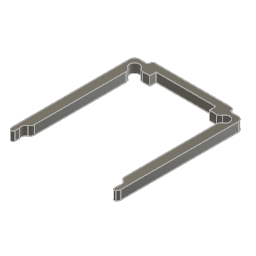
Screen Spacer v4 (Autodesk Fusion 360 design; units mm, degrees)
Autodesk Fusion 360 part; units mm, degrees
sketch "Sketch1" plane through (0, 0, 0) normal (0, 1, 0) x (1, 0, 0)
  line L0 (0, 0) -> (20, 0) construction
  line L1 (20, 0) -> (20, 24) construction
  line L2 (20, 24) -> (0, 24) construction
  line L3 (0, 24) -> (0, 0) construction
  circle A0 centre (0, 24) radius 1.1
  circle A1 centre (20, 24) radius 1.1
  circle A2 centre (20, 0) radius 1.1
  circle A3 centre (0, 0) radius 1.1
  line L4 (-2, 26) -> (22, 26)
  line L5 (22, 26) -> (22, -2)
  line L6 (22, -2) -> (-2, -2)
  line L7 (-2, -2) -> (-2, 26)
  line L8 (0, 24) -> (20, 24)
  line L9 (20, 24) -> (20, 0)
  line L10 (20, 0) -> (0, 0)
  line L11 (0, 0) -> (0, 24)
  dimension "d1" = 24
  dimension "d2" = 20
  dimension "d3" = 2.2
  dimension "d4" = 2
  dimension "d5" = 2
  dimension "d6" = 2
  dimension "d7" = 2
  constraint horizontal L0
  constraint vertical L1
  constraint horizontal L2
  constraint vertical L3
  constraint coincident L0.start L3.end
  constraint coincident L2.end L3.start
  constraint coincident L1.end L2.start
  constraint coincident L0.end L1.start
  constraint equal A0 A3
  constraint equal A0 A1
  constraint equal A1 A2
  constraint horizontal L4
  constraint vertical L5
  constraint horizontal L6
  constraint vertical L7
  constraint horizontal L8
  constraint vertical L9
  constraint horizontal L10
  constraint vertical L11
  measures "d1" distance of L0.start L2.end
  measures "d2" distance of L1.end L2.end
  measures "d3" diameter of A0
  measures "d4" distance of L2 L4
  measures "d5" distance of L1 L5
  measures "d6" distance of L0 L6
  measures "d7" distance of L3 L7
extrude "Extrude1" add sketch "Sketch1" along normal blind 2
fillet "Fillet1" radius 1 8 edges at (1.1, 1, -24) (0, 1, -22.9) (0, 1, -1.1) (18.9, 1, -24) (1.1, 1, 0) (20, 1, -22.9) (20, 1, -1.1) (18.9, 1, 0)
fillet "Fillet2" radius 1 4 edges at (-2, 1, -26) (-2, 1, 2) (22, 1, 2) (22, 1, -26)
extrude "Extrude2" cut 1 faces at (13.6667, 0.6667, 2) along direction (0, 0, -1) up to surface (2 mm away)
fillet "Fillet3" radius 0.4 2 edges at (-1, 1, 2) (21, 1, 2)
sketch "Sketch2" plane through (0, 2, 0) normal (0, 1, 0) x (-1, 0, 0)
  arc A0 (-21, 1.4472) -> (-21.6667, 1.7454) centre (-21.4, 1.4472) ccw
  arc A1 (-21.6667, 1.7454) -> (-22, 1) centre (-21, 1) ccw
  line L0 (-22, 1) -> (-22, -25)
  arc A2 (-22, -25) -> (-21, -26) centre (-21, -25) ccw
  line L1 (-21, -26) -> (1, -26)
  arc A3 (1, -26) -> (2, -25) centre (1, -25) ccw
  line L2 (2, -25) -> (2, 1)
  arc A4 (2, 1) -> (1.6667, 1.7454) centre (1, 1) ccw
  arc A5 (1.6667, 1.7454) -> (1, 1.4472) centre (1.4, 1.4472) ccw
  line L3 (1, 1.4472) -> (1, 0.4583)
  arc A6 (0.5238, -0.9673) -> (1, 0.4583) centre (0, 0) ccw
  arc A7 (0.5238, -0.9673) -> (0, -1.8466) centre (1, -1.8466) ccw
  line L4 (0, -1.8466) -> (0, -22.1534)
  arc A8 (0, -22.1534) -> (0.5238, -23.0327) centre (1, -22.1534) ccw
  arc A9 (-0.9673, -24.5238) -> (0.5238, -23.0327) centre (0, -24) ccw
  arc A10 (-0.9673, -24.5238) -> (-1.8466, -24) centre (-1.8466, -25) ccw
  line L5 (-1.8466, -24) -> (-18.1534, -24)
  arc A11 (-18.1534, -24) -> (-19.0327, -24.5238) centre (-18.1534, -25) ccw
  arc A12 (-20.5238, -23.0327) -> (-19.0327, -24.5238) centre (-20, -24) ccw
  arc A13 (-20.5238, -23.0327) -> (-20, -22.1534) centre (-21, -22.1534) ccw
  line L6 (-20, -22.1534) -> (-20, -1.8466)
  arc A14 (-20, -1.8466) -> (-20.5238, -0.9673) centre (-21, -1.8466) ccw
  arc A15 (-21, 0.4583) -> (-20.5238, -0.9673) centre (-20, 0) ccw
  line L7 (-21, 0.4583) -> (-21, 1.4472)
  line L8 (-3.4, -24) -> (-16.6, -24)
  line L9 (-16.6, -24) -> (-16.6, -25.4)
  line L10 (-16.6, -25.4) -> (-3.4, -25.4)
  line L11 (-3.4, -25.4) -> (-3.4, -24)
  line L12 (-1, -26) -> (-1, -27)
  line L13 (-1, -27) -> (-19, -27)
  line L14 (-19, -27) -> (-19, -26)
  line L15 (-1, -26) -> (-19, -26)
  dimension "d18" = 1.4
  dimension "d19" = 13.2
  dimension "d20" = 1
  dimension "d21" = 18
  constraint horizontal L8
  constraint vertical L9
  constraint horizontal L10
  constraint vertical L11
  constraint coincident L5 L8.start
  constraint midpoint L5 L8
  constraint coincident L1 L12.start
  constraint perpendicular L1 L12
  constraint perpendicular L12 L13
  constraint coincident L1 L14.end
  constraint perpendicular L1 L14
  constraint midpoint L1 L15
  measures "d18" distance of L8.end L9.end
  measures "d19" distance of L9.end L10.end
  measures "d20" distance of L12.start L12.end
  measures "d21" distance of L12.end L13.end
extrude "Extrude3" cut sketch "Sketch2" against normal up to surface (2 mm away) contours L5 L8 L9 L10 L11
extrude "Extrude4" add sketch "Sketch2" against normal up to surface (2 mm away) contours L1 L12 L13 L14 L15
fillet "Fillet5" radius 0.5 4 edges at (1, 1, -26) (1, 1, -27) (19, 1, -27) (19, 1, -26)
